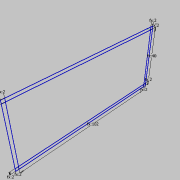
# Autodesk Inventor part: boitier_laser
Saved by Autodesk Inventor 2022 (Build 260153000, 153)
## iProperties
Created: 2021-11-29
Part Number: boitier_laser
Material: Generic
Document SubType Name: Modeling
Designer: jojo6
Density: 1 g/cm^3
Appearance: Default
Author: jojo6
Autodesk Inventor part; units mm, degrees
ref_plane "YZ Plane" through (0, 0, 0) normal (1, 0, 0) x (0, 1, 0)
ref_plane "XZ Plane" through (0, 0, 0) normal (0, 1, 0) x (-1, 0, 0)
ref_plane "XY Plane" through (0, 0, 0) normal (0, 0, 1) x (1, 0, 0)
sketch "Sketch1" plane through (0, 0, 0) normal (0, 1, 0) x (-1, 0, 0)
  line L0 (0, 0) -> (47, 0)
  line L1 (47, 0) -> (47, 102)
  line L2 (47, 102) -> (0, 102)
  line L3 (0, 102) -> (0, 0)
  line L4 (47, 0) -> (49, 0)
  line L5 (49, 0) -> (49, -2)
  line L6 (49, -2) -> (47, -2)
  line L7 (47, -2) -> (47, 0)
  line L8 (47, 102) -> (49, 102)
  line L9 (49, 102) -> (49, 104)
  line L10 (49, 104) -> (47, 104)
  line L11 (47, 104) -> (47, 102)
  line L12 (0, 102) -> (-2, 102)
  line L13 (-2, 102) -> (-2, 104)
  line L14 (-2, 104) -> (0, 104)
  line L15 (0, 104) -> (0, 102)
  line L16 (0, 0) -> (-2, 0)
  line L17 (-2, 0) -> (-2, -2)
  line L18 (-2, -2) -> (0, -2)
  line L19 (0, -2) -> (0, 0)
  line L20 (47, -2) -> (0, -2)
  line L21 (-2, 0) -> (-2, 102)
  line L22 (0, 104) -> (47, 104)
  line L23 (49, 102) -> (49, 0)
  line L24 (23.5, 102) -> (23.5, 90.5)
  line L25 (23.5, 90.5) -> (23.5, 88)
  circle A0 centre (23.5, 88) radius 2.5
  line L26 (47, 51) -> (0, 51)
  circle A1 centre (23.5, 14) radius 2.5
  dimension "d14" = 47
  dimension "d15" = 102
  dimension "d16" = 2
  dimension "d17" = 2
  dimension "d18" = 2
  dimension "d19" = 2
  dimension "d20" = 2
  dimension "d21" = 2
  dimension "d22" = 2
  dimension "d23" = 2
  dimension "d28" = 11.5
  dimension "d29" = 2.5
  constraints: 54 end point, 10 parallel, 5 horizontal, 5 perpendicular, 3 midpoint, 2 vertical, 1 centre point, 1 coincident, 1 symmetric about line, 1 vertical alignment, 3 other
  measures "d14" distance of L2.end L1.end
  measures "d15" distance of L1.end L0.end
  measures "d16" distance of L5.end L6.end
  measures "d17" distance of L4.end L5.end
  measures "d18" distance of L10.end L9.end
  measures "d19" distance of L9.end L8.end
  measures "d20" distance of L13.end L14.end
  measures "d21" distance of L12.end L13.end
  measures "d22" distance of L18.end L17.end
  measures "d23" distance of L17.end L16.end
  measures "d28" distance of L24.start L24.end
  measures "d29" distance of L24.end L25.end
sketch "Sketch2" plane through (0, 0, 0) normal (1, 0, 0) x (0, 1, 0)
  point P0 (0, 0)
extrude "Extrusion1" add sketch "Sketch1" along normal blind 2
sketch "Sketch3" plane through (2, 0, 104) normal (1, 0, 0) x (0, 0, -1)
  point P0 (104, 0)
sketch "Sketch4" plane through (2, 0, 104) normal (1, 0, 0) x (0, 0, -1)
  line L0 (106, 0) -> (0, 0) projected
  line L1 (0, 0) -> (2, 0)
  line L2 (2, 0) -> (2, 2)
  line L3 (2, 2) -> (0, 2)
  line L4 (0, 2) -> (0, 0)
  line L5 (2, 0) -> (104, 0)
  line L6 (104, 0) -> (104, -40)
  line L7 (104, -40) -> (2, -40)
  line L8 (2, -40) -> (2, 0)
  line L9 (2, -40) -> (0, -40)
  line L10 (0, -40) -> (0, -42)
  line L11 (0, -42) -> (2, -42)
  line L12 (2, -42) -> (2, -40)
  line L13 (104, -40) -> (106, -40)
  line L14 (106, -40) -> (106, -42)
  line L15 (106, -42) -> (104, -42)
  line L16 (104, -42) -> (104, -40)
  line L17 (104, 0) -> (106, 0)
  line L18 (106, 0) -> (106, 2)
  line L19 (106, 2) -> (104, 2)
  line L20 (104, 2) -> (104, 0)
  line L21 (0, 0) -> (0, -40)
  line L22 (2, -42) -> (104, -42)
  line L23 (106, -40) -> (106, 0)
  line L24 (2, 2) -> (104, 2)
  dimension "d33" = 2
  dimension "d34" = 2
  dimension "d35" = 102
  dimension "d36" = 40
  dimension "d37" = 2
  dimension "d38" = 2
  dimension "d39" = 2
  dimension "d40" = 2
  dimension "d41" = 2
  dimension "d42" = 2
  constraints: 48 end point, 10 parallel, 5 horizontal, 5 perpendicular
  measures "d33" distance of L3.end L2.end
  measures "d34" distance of L2.end L1.end
  measures "d35" distance of L6.end L7.end
  measures "d36" distance of L5.end L6.end
  measures "d37" distance of L11.end L10.end
  measures "d38" distance of L10.end L9.end
  measures "d39" distance of L14.end L15.end
  measures "d40" distance of L13.end L14.end
  measures "d41" distance of L19.end L18.end
  measures "d42" distance of L18.end L17.end
equation "\"d14\" = largeur_ins"
equation "\"d15\" = longueur_ins"
equation "\"d16\" = epaisseur"
equation "\"d17\" = epaisseur"
equation "\"d18\" = epaisseur"
equation "\"d19\" = epaisseur"
equation "\"d20\" = epaisseur"
equation "\"d21\" = epaisseur"
equation "\"d22\" = epaisseur"
equation "\"d23\" = epaisseur"
equation "\"d31\" = epaisseur"
equation "\"d33\" = epaisseur"
equation "\"d34\" = epaisseur"
equation "\"d35\" = longueur_ins"
equation "\"d36\" = hauteur_inside"
equation "\"d37\" = epaisseur"
equation "\"d38\" = epaisseur"
equation "\"d39\" = epaisseur"
equation "\"d40\" = epaisseur"
equation "\"d41\" = epaisseur"
equation "\"d42\" = epaisseur"
equation "\"epaisseur\" = 2"
equation "\"largeur_ins\" = 47"
equation "\"longueur_ins\" = 102"
equation "\"dist_laser\" = 69"
equation "\"hauteur_inside\" = 40"
body "Solid1"
